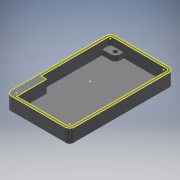
# Autodesk Inventor part: Case_3_inferior
Saved by Autodesk Inventor 2019 (Build 230136000, 136)
## iProperties
Created: 2018-11-27
Part Number: Case_3_inferior
Material: Steel, Mild, Welded
Document SubType Name: Modeling
Designer: cadcae
Density: 7.85 g/cm^3
Appearance: Smooth - Medium Gray
Author: cadcae
Autodesk Inventor part; units mm, degrees
ref_plane "YZ Plane" through (0, 0, 0) normal (1, 0, 0) x (0, 1, 0)
ref_plane "XZ Plane" through (0, 0, 0) normal (0, 1, 0) x (-1, 0, 0)
ref_plane "XY Plane" through (0, 0, 0) normal (0, 0, 1) x (1, 0, 0)
sketch "Sketch1" plane through (0, 0, 0) normal (0, 1, 0) x (-1, 0, 0)
  line L0 (-28.525, 48.63) -> (28.525, 48.63)
  line L1 (28.525, 48.63) -> (28.525, -48.63)
  line L2 (28.525, -48.63) -> (-28.525, -48.63)
  line L3 (-28.525, -48.63) -> (-28.525, 48.63)
  line L4 (-28.525, 48.63) -> (28.525, -48.63) construction
  line L5 (28.525, 48.63) -> (-28.525, -48.63) construction
  line L6 (29.025, -49.13) -> (29.025, 49.13)
  line L7 (29.025, 49.13) -> (-29.025, 49.13)
  line L8 (-29.025, 49.13) -> (-29.025, -49.13)
  line L9 (-29.025, -49.13) -> (29.025, -49.13)
  line L10 (31.425, 51.53) -> (31.425, -51.53)
  line L11 (31.425, -51.53) -> (-31.425, -51.53)
  line L12 (-31.425, -51.53) -> (-31.425, 51.53)
  line L13 (-31.425, 51.53) -> (31.425, 51.53)
  point P0 (0, 0)
  dimension "d0" = 97.26
  dimension "d1" = 57.05
  dimension "d2" = 0.5
  dimension "d3" = 2.4
  constraints: 28 end point, 6 parallel, 3 perpendicular, 2 midpoint, 1 horizontal, 6 other
  measures "d0" distance of L0.end L1.end
  measures "d1" distance of L1.end L2.end
  measures "d2" distance between parallel lines of L1 L6
  measures "d3" distance between parallel lines of L6 L10
extrude "Extrusion1" add sketch "Sketch1" against normal blind 14.87 contours L0 L1 L2 L3 | L9 L8 L7 L6 | L10 L11 L12 L13
fillet "Fillet2" radius 5 4 edges at (-31.425, -7.435, -51.53) (-31.425, -7.435, 51.53) (31.425, -7.435, 51.53) (31.425, -7.435, -51.53)
shell "Shell1" thickness 2.4 removed faces 1 at (10.475, 0, 15.51)
chamfer "Chamfer1" distance 2 angle 45 4 edges at (31.425, -14.87, 0) (0, -14.87, 51.53) (-31.425, -14.87, 0) (0, -14.87, -51.53)
sketch "Sketch7" plane through (-26.425, -12.47, -49.13) normal (0, 1, 0) x (1, 0, 0)
  arc A0 (55.45, -2.6) -> (52.85, 0) centre (52.85, -2.6) ccw projected
  line L0 (0, 0) -> (52.85, 0) projected
  arc A1 (0, 0) -> (-2.6, -2.6) centre (0, -2.6) ccw projected
  line L1 (-2.6, -95.66) -> (-2.6, -2.6) projected
  arc A2 (-2.6, -95.66) -> (0, -98.26) centre (0, -95.66) ccw projected
  line L2 (52.85, -98.26) -> (0, -98.26) projected
  arc A3 (52.85, -98.26) -> (55.45, -95.66) centre (52.85, -95.66) ccw projected
  line L3 (55.45, -2.6) -> (55.45, -95.66) projected
  line L4 (4.88, -97.76) -> (52.95, -97.76) construction
  line L5 (54.95, -95.76) -> (54.95, -2.5) construction
  line L6 (52.95, -0.5) -> (4.88, -0.5) construction
  line L7 (2.88, -2.5) -> (2.88, -95.76) construction
  arc A4 (2.88, -95.76) -> (4.88, -97.76) centre (4.88, -95.76) ccw construction
  arc A5 (4.88, -0.5) -> (2.88, -2.5) centre (4.88, -2.5) ccw construction
  arc A6 (54.95, -2.5) -> (52.95, -0.5) centre (52.95, -2.5) ccw construction
  arc A7 (52.95, -97.76) -> (54.95, -95.76) centre (52.95, -95.76) ccw construction
  line L8 (2.88, -68.66) -> (-2.1, -68.66)
  line L9 (-2.1, -68.66) -> (-2.1, -50.66)
  line L10 (-2.1, -50.66) -> (2.88, -50.66)
  line L11 (-2.1, -68.66) -> (-2.6, -68.66)
  circle A8 centre (5.88, -94.76) radius 1.8 construction
  line L12 (2.88, -89.96) -> (5.88, -89.96)
  arc A9 (10.68, -94.76) -> (5.88, -89.96) centre (5.88, -94.76) ccw
  line L13 (10.68, -94.76) -> (10.68, -98.26)
  line L14 (10.68, -98.26) -> (0, -98.26)
  line L15 (-2.6, -95.66) -> (-2.6, -68.66)
  arc A10 (-2.6, -95.66) -> (0, -98.26) centre (0, -95.66) ccw
  circle A11 centre (5.88, -3.5) radius 1.8 construction
  line L16 (10.68, 0) -> (10.68, -3.5)
  line L17 (-2.6, -8.3) -> (5.88, -8.3)
  arc A12 (5.88, -8.3) -> (10.68, -3.5) centre (5.88, -3.5) ccw
  line L18 (-2.6, -8.3) -> (-2.6, -2.6)
  line L19 (10.68, 0) -> (0, 0)
  arc A13 (0, 0) -> (-2.6, -2.6) centre (0, -2.6) ccw
  line L20 (2.88, -89.96) -> (2.88, -68.66)
  line L21 (48.45, -98.26) -> (55.45, -91.26)
  line L22 (48.45, -98.26) -> (52.85, -98.26)
  line L23 (55.45, -91.26) -> (55.45, -95.66)
  arc A14 (52.85, -98.26) -> (55.45, -95.66) centre (52.85, -95.66) ccw
  circle A15 centre (51.95, -3.5) radius 1.8 construction
  line L24 (55.45, -8.3) -> (51.95, -8.3)
  line L25 (47.15, 0) -> (47.15, -3.5)
  arc A16 (47.15, -3.5) -> (51.95, -8.3) centre (51.95, -3.5) ccw
  line L26 (55.45, -8.3) -> (55.45, -2.6)
  line L27 (55.85, -95.66) -> (55.85, -2.6) projected
  line L28 (47.15, 0) -> (52.85, 0)
  arc A17 (55.45, -2.6) -> (52.85, 0) centre (52.85, -2.6) ccw
  point P0 (26.425, -49.13)
  point P1 (54.95, -0.5)
  point P2 (54.95, -97.76)
  point P3 (2.88, -0.5)
  dimension "d43" = 52.07
  dimension "d44" = 97.26
  dimension "d45" = 0.5
  dimension "d46" = 0.5
  dimension "d47" = 2
  dimension "d48" = 18
  dimension "d49" = 4.98
  dimension "d50" = 29.1
  dimension "d51" = 3.6
  dimension "d52" = 3
  dimension "d53" = 3
  dimension "d54" = 3
  dimension "d55" = 3.6
  dimension "d56" = 3
  dimension "d57" = 3
  dimension "d58" = 45
  dimension "d59" = 7
  dimension "d60" = 3.6
  dimension "d61" = 3
  dimension "d62" = 3
  constraints: 48 end point, 22 point on circle, 18 tangent, 17 point on line, 14 centre point, 6 coincident, 6 horizontal, 5 collinear, 4 perpendicular, 4 vertical, 3 equal radius, 3 parallel, 1 concentric, 1 horizontal alignment, 1 vertical alignment
  measures "d43" distance of point (2.88, -0.5) point (54.95, -0.5)
  measures "d44" distance of point (54.95, -0.5) point (54.95, -97.76)
  measures "d45" distance between parallel lines of L3 L5
  measures "d46" distance between parallel lines of L2 L4
  measures "d47" radius of A4
  measures "d48" distance of L8.end L9.end
  measures "d49" distance of L8.start L8.end
  measures "d50" distance between parallel lines of L4 L8
  measures "d51" diameter of A8
  measures "d52" distance from line of A8.centre L4
  measures "d53" distance from line of L7 A8.centre
  measures "d54" radial gap between concentric circles of A9 A8
  measures "d55" diameter of A11
  measures "d56" distance from line of L6 A11.centre
  measures "d57" radial gap between concentric circles of A12 A11
  measures "d58" angle of L5 L21
  measures "d59" distance from line of L3 L21.start
  measures "d60" diameter of A15
  measures "d61" distance from line of L5 A15.centre
  measures "d62" radial gap between concentric circles of A16 A15
extrude "Extrusion7" add sketch "Sketch7" along normal blind 4.9 contours L3 L24 A16 L25 L0 A0 | L3 A3 L2 L21 | L16 A12 L17 L1 A1 L0 | L2 A2 L1 L11 L8 L20 L12 A9 L13
sketch "Sketch8" plane through (-26.425, -7.57, -49.13) normal (0, 1, 0) x (1, 0, 0)
  arc A0 (10.68, -94.76) -> (5.88, -89.96) centre (5.88, -94.76) ccw projected
  circle A1 centre (5.88, -94.76) radius 1.8
  circle A2 centre (5.88, -3.5) radius 1.8
  circle A3 centre (51.95, -3.5) radius 1.8
  arc A4 (5.88, -8.3) -> (10.68, -3.5) centre (5.88, -3.5) ccw projected
  arc A5 (47.15, -3.5) -> (51.95, -8.3) centre (51.95, -3.5) ccw projected
  arc A6 (-2.6, -95.66) -> (0, -98.26) centre (0, -95.66) ccw projected
  line L0 (10.68, -98.26) -> (0, -98.26) projected
  line L1 (10.68, -98.26) -> (10.68, -94.76) projected
  arc A7 (10.68, -94.76) -> (5.88, -89.96) centre (5.88, -94.76) ccw projected
  line L2 (5.88, -89.96) -> (2.88, -89.96) projected
  line L3 (2.88, -89.96) -> (2.88, -68.66) projected
  line L4 (2.88, -68.66) -> (-2.6, -68.66) projected
  line L5 (-2.6, -95.66) -> (-2.6, -68.66) projected
  line L6 (2.88, -89.96) -> (5.88, -89.96) projected
  line L7 (2.88, -89.96) -> (2.88, -98.26)
  line L8 (10.68, -98.26) -> (0, -98.26) projected
  line L9 (2.88, -98.26) -> (0, -98.26)
  point P0 (26.425, -49.13)
  dimension "d65" = 3.6
  constraints: 4 end point, 3 centre point, 3 coincident, 2 equal radius, 1 collinear, 1 perpendicular, 1 point on line
  measures "d65" diameter of A1
extrude "Extrusion8" cut sketch "Sketch8" against normal blind 2.5 contours A1 | A2 | A3
extrude "Extrusion9" add sketch "Sketch8" along normal up to surface (7.57 mm away) contours L7 L0 A6 L5 L4 L3
sketch "Sketch9" plane through (0, 0, 0) normal (0, 1, 0) x (1, 0, 0)
  arc A0 (29.025, 46.53) -> (26.425, 49.13) centre (26.425, 46.53) ccw projected
  line L0 (29.025, 46.53) -> (29.025, -46.53) projected
  arc A1 (26.425, -49.13) -> (29.025, -46.53) centre (26.425, -46.53) ccw projected
  line L1 (26.425, -49.13) -> (-23.545, -49.13) projected
  line L2 (-23.545, -49.13) -> (-23.545, -19.53) projected
  line L3 (-23.545, -19.53) -> (-29.025, -19.53) projected
  line L4 (-29.025, -19.53) -> (-29.025, 46.53) projected
  arc A2 (-26.425, 49.13) -> (-29.025, 46.53) centre (-26.425, 46.53) ccw projected
  line L5 (-26.425, 49.13) -> (26.425, 49.13) projected
  arc A3 (31.425, 46.53) -> (26.425, 51.53) centre (26.425, 46.53) ccw projected
  line L6 (-26.425, 51.53) -> (26.425, 51.53) projected
  arc A4 (-26.425, 51.53) -> (-31.425, 46.53) centre (-26.425, 46.53) ccw projected
  line L7 (-31.425, -46.53) -> (-31.425, 46.53) projected
  arc A5 (-31.425, -46.53) -> (-26.425, -51.53) centre (-26.425, -46.53) ccw projected
  line L8 (26.425, -51.53) -> (-26.425, -51.53) projected
  arc A6 (26.425, -51.53) -> (31.425, -46.53) centre (26.425, -46.53) ccw projected
  line L9 (31.425, 46.53) -> (31.425, -46.53) projected
  point P0 (0, 0)
equation "\"d56\" = d52"
equation "\"d61\" = d53"
body "Solid1"
